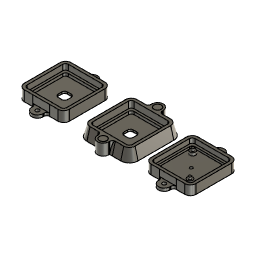
reader_scanner_case_v3 (Autodesk Fusion 360 design; units mm, degrees)
Autodesk Fusion 360 part; units mm, degrees
note: some values were not read from the file. Chosen so that the rebuilt part matches the saved one: which pieces of a blend or face edit are solid. Set by a fixed rule: which sketch regions a step uses; which face or edge a step refers to.
sketch "Sketch1" plane through (0, 0, 0) normal (0, 0, 1) x (1, 0, 0)
  line L0 (18, -22) -> (-18, -22)
  line L1 (-21, -19) -> (-21, 19)
  line L2 (-18, 22) -> (18, 22)
  line L3 (21, 19) -> (21, -19)
  line L4 (21, -22) -> (-21, 22) construction
  line L5 (-21, -22) -> (21, 22) construction
  arc A0 (-18, 22) -> (-21, 19) centre (-18, 19) ccw
  arc A1 (21, 19) -> (18, 22) centre (18, 19) ccw
  arc A2 (18, -22) -> (21, -19) centre (18, -19) ccw
  arc A3 (-21, -19) -> (-18, -22) centre (-18, -19) ccw
  arc A4 (-24, -19) -> (-18, -25) centre (-18, -19) ccw
  line L6 (-24, -19) -> (-24, 19)
  arc A5 (-18, 25) -> (-24, 19) centre (-18, 19) ccw
  arc A6 (24, 19) -> (18, 25) centre (18, 19) ccw
  line L7 (24, 19) -> (24, -19)
  arc A7 (18, -25) -> (24, -19) centre (18, -19) ccw
  line L8 (-2, 5) -> (2, 5)
  line L9 (5, 2) -> (5, -2)
  line L10 (2, -5) -> (-2, -5)
  line L11 (-5, -2) -> (-5, 2)
  arc A8 (-2, 5) -> (-5, 2) centre (-2, 2) ccw
  arc A9 (5, 2) -> (2, 5) centre (2, 2) ccw
  arc A10 (2, -5) -> (5, -2) centre (2, -2) ccw
  arc A11 (-5, -2) -> (-2, -5) centre (-2, -2) ccw
  circle A12 centre (14.2, -15.5) radius 3.125
  circle A13 centre (-14.2, 15.5) radius 3.125
  line L12 (0, 0) -> (0, 20)
  circle A14 centre (14.2, 15.5) radius 3.125
  circle A15 centre (-14.2, -15.5) radius 3.125
  circle A16 centre (0, -29) radius 2
  circle A17 centre (0, 29) radius 2
  line L13 (-6, 29) -> (-6, 28)
  line L14 (6, 29) -> (6, 28)
  line L15 (6, -29) -> (6, -28)
  line L16 (-6, -29) -> (-6, -28)
  arc A18 (6, 29) -> (-6, 29) centre (0, 29) ccw
  arc A19 (-6, -29) -> (6, -29) centre (0, -29) ccw
  line L17 (18, -25) -> (9, -25)
  line L18 (-9, -25) -> (-18, -25)
  line L19 (9, -25) -> (-9, -25)
  line L20 (-18, 25) -> (-9, 25)
  line L21 (9, 25) -> (18, 25)
  line L22 (-9, 25) -> (9, 25)
  arc A20 (6, 28) -> (9, 25) centre (9, 28) ccw
  arc A21 (-9, 25) -> (-6, 28) centre (-9, 28) ccw
  arc A22 (9, -25) -> (6, -28) centre (9, -28) ccw
  arc A23 (-6, -28) -> (-9, -25) centre (-9, -28) ccw
  line L23 (18.5, 16.5) -> (18.5, -16.5)
  line L24 (-15.5, 19.5) -> (15.5, 19.5)
  line L25 (-18.5, -16.5) -> (-18.5, 16.5)
  line L26 (15.5, -19.5) -> (-15.5, -19.5)
  arc A24 (15.5, -19.5) -> (18.5, -16.5) centre (15.5, -16.5) ccw
  arc A25 (-18.5, -16.5) -> (-15.5, -19.5) centre (-15.5, -16.5) ccw
  arc A26 (-15.5, 19.5) -> (-18.5, 16.5) centre (-15.5, 16.5) ccw
  arc A27 (18.5, 16.5) -> (15.5, 19.5) centre (15.5, 16.5) ccw
  circle A28 centre (0, -29) radius 4
  circle A29 centre (0, 29) radius 4
  circle A30 centre (0, -29) radius 3.85
  circle A31 centre (0, 29) radius 3.85
  dimension "d1" = 42
  dimension "d2" = 44
  dimension "d4" = 3
  dimension "d5" = 3
  dimension "d6" = 3
  dimension "d13" = 6.25
  dimension "d14" = 6.25
  dimension "d15" = 3
  dimension "d16" = 3
  dimension "d17" = 3
  dimension "d18" = 3
  dimension "d28" = 3
  dimension "d29" = 3
  dimension "d30" = 3
  dimension "d31" = 3
  dimension "d34" = 4
  dimension "d79" = 7.7
  dimension "d80" = 7.7
  constraint horizontal L0
  constraint perpendicular L0 L1
  constraint parallel L0 L2
  constraint parallel L1 L3
  constraint coincident L4 L12.start
  constraint coincident L5 L12.start
  constraint coincident L12.start origin
  constraint coincident L4.end L1
  constraint coincident L4.end L2
  constraint tangent L1 A0
  constraint tangent L2 A0
  constraint coincident L5.end L2
  constraint coincident L5.end L3
  constraint tangent L2 A1
  constraint tangent L3 A1
  constraint equal A0 A1
  constraint coincident L4.start L3
  constraint coincident L4.start L0
  constraint tangent L3 A2
  constraint tangent L0 A2
  constraint equal A0 A2
  constraint coincident L5.start L0
  constraint coincident L5.start L1
  constraint tangent L0 A3
  constraint tangent L1 A3
  constraint equal A0 A3
  constraint horizontal L8
  constraint vertical L9
  constraint horizontal L10
  constraint vertical L11
  constraint tangent L8 A8
  constraint tangent L11 A8
  constraint tangent L8 A9
  constraint tangent L9 A9
  constraint equal A8 A9
  constraint tangent L9 A10
  constraint tangent L10 A10
  constraint equal A8 A10
  constraint tangent L10 A11
  constraint tangent L11 A11
  constraint perpendicular L12 L20
  constraint symmetric A12 L12 A15
  constraint symmetric A13 L12 A14
  constraint tangent L13 A18
  constraint perpendicular L13 L20
  constraint tangent L14 A18
  constraint perpendicular L14 L20
  constraint tangent L15 A19
  constraint perpendicular L15 L17
  constraint tangent L16 A19
  constraint perpendicular L16 L17
  constraint concentric A3 A4
  constraint concentric A0 A5
  constraint concentric A1 A6
  constraint concentric A2 A7
  constraint tangent A4 L17
  constraint tangent A7 L17
  constraint tangent A6 L7
  constraint tangent A4 L6
  constraint tangent L7 A7
  constraint tangent L6 A5
  constraint tangent A6 L20
  constraint tangent A5 L20
  constraint tangent L14 A20
  constraint tangent L21 A20
  constraint tangent L13 A21
  constraint tangent L20 A21
  constraint tangent L15 A22
  constraint tangent L17 A22
  constraint tangent L16 A23
  constraint tangent L18 A23
  constraint tangent L23 A24
  constraint tangent L26 A24
  constraint tangent L26 A25
  constraint tangent L25 A25
  constraint tangent L24 A26
  constraint tangent L25 A26
  constraint tangent L23 A27
  constraint tangent L24 A27
  constraint concentric A19 A28
  constraint tangent L19 A28
  constraint concentric A17 A29
  constraint tangent L22 A29
  constraint concentric A28 A30
  constraint concentric A17 A31
  measures "d1" distance of L4.end L5.end
  measures "d2" distance of L5.start L4.end
  measures "d4" radius of A0
  measures "d5" radius of A8
  measures "d6" radius of A11
  measures "d13" diameter of A12
  measures "d14" diameter of A13
  measures "d15" radius of A20
  measures "d16" radius of A21
  measures "d17" radius of A22
  measures "d18" radius of A23
  measures "d28" radius of A24
  measures "d29" radius of A25
  measures "d30" radius of A26
  measures "d31" radius of A27
  measures "d34" diameter of A17
  measures "d79" diameter of A30
  measures "d80" diameter of A31
extrude "Extrude1" add sketch "Sketch1" along normal blind 10 contours A4 L6 A5 A6 L7 A7 L17 L18 L19 L20 L21 L22 makes body 1
extrude "Extrude2" add sketch "Sketch1" along normal blind 2 contours L0 L1 L2 L3 A0 A1 A2 A3 | L23 L24 L25 L26 A24 A25 A26 A27 bodies 1
extrude "Extrude3" add sketch "Sketch1" along normal blind 3 contours A28 | L15 L16 A19 L19 A22 A23 | A29 | L13 L14 A18 L22 A20 A21 | A30 | A31 bodies 1
extrude "Extrude4" add sketch "Sketch1" along normal blind 2 contours A12 | A13 | A14 | A15 bodies 1
extrude "Extrude5" add sketch "Sketch1" along normal blind 5 contours L0 L1 L2 L3 A0 A1 A2 A3 bodies 1
copy_body "CopyPasteBodies1" bodies 1 makes body 2
move_body "Move1" bodies 2 to x (1, 0, 0) y (0, 1, 0) z (0, 0, 1) at (65, 0, 0)
sketch "Sketch2" plane through (0, 0, 2) normal (0, 0, 1) x (-1, 0, 0)
  line L0 (-83.5, 16.5) -> (-83.5, -16.5)
  arc A0 (-83.5, -16.5) -> (-80.5, -19.5) centre (-80.5, -16.5) ccw
  line L1 (-80.5, -19.5) -> (-49.5, -19.5)
  arc A1 (-49.5, -19.5) -> (-46.5, -16.5) centre (-49.5, -16.5) ccw
  line L2 (-46.5, -16.5) -> (-46.5, 16.5)
  arc A2 (-46.5, 16.5) -> (-49.5, 19.5) centre (-49.5, 16.5) ccw
  line L3 (-49.5, 19.5) -> (-80.5, 19.5)
  arc A3 (-80.5, 19.5) -> (-83.5, 16.5) centre (-80.5, 16.5) ccw
  arc A4 (-63, -5) -> (-60, -2) centre (-63, -2) ccw
  line L4 (-63, -5) -> (-67, -5)
  arc A5 (-70, -2) -> (-67, -5) centre (-67, -2) ccw
  line L5 (-70, -2) -> (-70, 2)
  arc A6 (-67, 5) -> (-70, 2) centre (-67, 2) ccw
  line L6 (-67, 5) -> (-63, 5)
  arc A7 (-60, 2) -> (-63, 5) centre (-63, 2) ccw
  line L7 (-60, 2) -> (-60, -2)
  circle A8 centre (-52.7, -13.8) radius 1.4
  circle A9 centre (-77.3, 13.8) radius 1.4
  circle A10 centre (-77.3, 13.8) radius 3
  circle A11 centre (-52.7, -13.8) radius 3
  circle A12 centre (-65, 0) radius 1.5
  arc A13 (-69.8, -2) -> (-67, -4.8) centre (-67, -2) ccw
  line L8 (-63, -4.8) -> (-67, -4.8)
  arc A14 (-63, -4.8) -> (-60.2, -2) centre (-63, -2) ccw
  line L9 (-60.2, 2) -> (-60.2, -2)
  arc A15 (-60.2, 2) -> (-63, 4.8) centre (-63, 2) ccw
  line L10 (-67, 4.8) -> (-63, 4.8)
  arc A16 (-67, 4.8) -> (-69.8, 2) centre (-67, 2) ccw
  line L11 (-69.8, -2) -> (-69.8, 2)
  line L12 (-46.7, -16.5) -> (-46.7, 16.5)
  arc A17 (-46.7, 16.5) -> (-49.5, 19.3) centre (-49.5, 16.5) ccw
  line L13 (-49.5, 19.3) -> (-80.5, 19.3)
  arc A18 (-80.5, 19.3) -> (-83.3, 16.5) centre (-80.5, 16.5) ccw
  line L14 (-83.3, 16.5) -> (-83.3, -16.5)
  arc A19 (-83.3, -16.5) -> (-80.5, -19.3) centre (-80.5, -16.5) ccw
  line L15 (-80.5, -19.3) -> (-49.5, -19.3)
  arc A20 (-49.5, -19.3) -> (-46.7, -16.5) centre (-49.5, -16.5) ccw
  line L16 (-65, 0) -> (-65, -14.5)
  line L17 (-65, 0) -> (-65, 14.5)
  point P0 (-65, 0)
  dimension "d37" = 2.8
  dimension "d38" = 2.8
  dimension "d39" = 6
  dimension "d40" = 6
  dimension "d41" = 3
  dimension "d42" = 0.2
  dimension "d43" = -0.2
  constraint concentric A8 A11
  constraint coincident P0 A12.centre
  constraint vertical L16
  constraint parallel L16 L17
  measures "d37" diameter of A8
  measures "d38" diameter of A9
  measures "d39" diameter of A10
  measures "d40" diameter of A11
  measures "d41" diameter of A12
extrude "Extrude6" add sketch "Sketch2" along normal blind 1 separate body contours A4 L4 L6 A7 L7 L8 A14 L9 A15 L10 L16 L17 | L4 A5 L5 A6 L6 A13 L8 L10 A16 L11 L16 L17 | A12 L8 A14 L9 A15 L10 L16 L17 | A12 A13 L8 L10 A16 L11 L16 L17 | L12 A17 L13 A18 L14 A19 L15 A20 makes body 3
extrude "Extrude7" add sketch "Sketch2" along normal blind 4 contours A10 bodies 3
extrude "Extrude8" add sketch "Sketch2" along normal blind 4 contours A11 bodies 3
extrude "Extrude9" add sketch "Sketch2" along normal blind 6 contours A8 | A9 bodies 3
extrude "Extrude10" add sketch "Sketch2" against normal blind 2 contours A12 L8 A14 L9 A15 L10 L16 L17 | A12 A13 L8 L10 A16 L11 L16 L17 bodies 3
extrude "Extrude11" add 2 faces at (50.2445, 13.949, 6) (76.6083, -16.1608, 6) along direction (0, 0, 1) blind 1 on bodies 3 bodies 3
extrude "Extrude12" add 2 faces at (52.9333, 13.3959, 8) (77.2651, -13.3965, 8) along direction (0, 0, 1) blind 1 on bodies 3 bodies 3
extrude "Extrude13" cut 2 faces at (50.2445, 13.949, 7) (76.6083, -16.1608, 7) along direction (0, 0, -1) blind 1 on bodies 3 bodies 3
extrude "Extrude14" cut 2 faces at (52.9333, 13.3959, 9) (77.2651, -13.3965, 9) along direction (0, 0, -1) blind 0.5 on bodies 3 bodies 3
move_body "Move2" bodies 1 to x (1, 0, 0) y (0, 1, 0) z (0, 0, 1) at (-70, 0, 0)
extrude "Extrude15" add 1 faces at (-73, -23, 10) along direction (0, 0, 1) blind 1 on bodies 1 bodies 1
extrude "Extrude16" add sketch "Sketch1" along normal blind 2 separate body contours A12 | A13 | A14 | A15 | L23 L24 L25 L26 A24 A25 A26 A27 makes body 4
extrude "Extrude17" add sketch "Sketch1" along normal blind 5 contours L0 L1 L2 L3 A0 A1 A2 A3 bodies 4
extrude "Extrude18" add sketch "Sketch1" along normal blind 11 contours A4 L6 A5 A6 L7 A7 L17 L18 L19 L20 L21 L22 bodies 4
extrude "Extrude19" add 1 faces at (-3, -23, 11) along direction (0, 0, 1) blind 1 on bodies 4 bodies 4
draft "Draft1" angle 15 neutral plane through (0, 0, 12) pull (0, 0, 1) 12 faces at (24, -6.3333, 8) (19.4146, 24.8309, 8) (15, 25, 8) (-3, 25, 8) (-15, 25, 4) (-23.8309, 20.4146, 8) (-24, 6.3333, 8) (-19.4146, -24.8309, 8) (-15, -25, 8) (3, -25, 8) (12, -25, 8) (23.8309, -20.4146, 8) on bodies 4
extrude "Extrude20" add sketch "Sketch1" along normal blind 12 contours A28 | L15 L16 A19 L19 A22 A23 | A29 | L13 L14 A18 L22 A20 A21 | A30 | A31 bodies 4
extrude "Extrude21" cut sketch "Sketch1" against normal blind 9 from surface at 12 contours A28 | A29 | A16 | A17 | A30 | A31 bodies 4
extrude "Extrude22" add sketch "Sketch1" against normal blind 3 from surface at 12 separate body contours A16 | A17 | A30 | A31 makes body 5 at (3.8452, -29.1919, 10) makes body 6 at (3.8452, 28.8081, 10)
